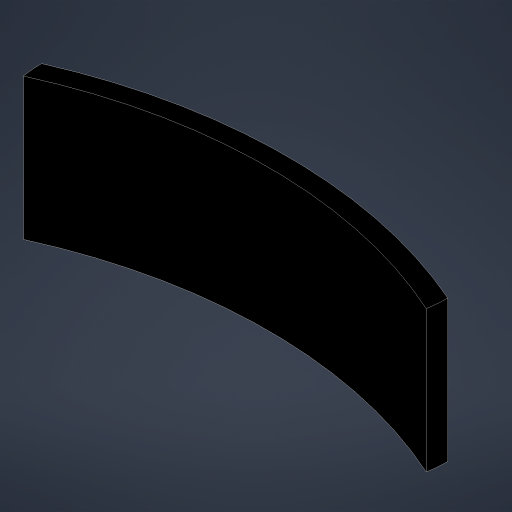
# Autodesk Inventor part: MettalringUnten_v3
Saved by Autodesk Inventor 2023.2 (Build 272271030, 271C)
## iProperties
Created: 2022-10-10
Part Number: MettalringUnten_v3
Material: Generic
Document SubType Name: Modeling
Designer: braun
Density: 1 g/cm^3
Appearance: Default
Author: braun
Autodesk Inventor part; units mm, degrees
ref_plane "YZ Plane" through (0, 0, 0) normal (1, 0, 0) x (0, 1, 0)
ref_plane "XZ Plane" through (0, 0, 0) normal (0, 1, 0) x (-1, 0, 0)
sketch "Sketch1" plane through (0, 0, 0) normal (0, 1, 0) x (-1, 0, 0)
  circle A0 centre (0, 0) radius 110 construction
  arc A1 (43.0581, -98.5) -> (-43.0581, -98.5) centre (0, 0) ccw
  line L0 (0, -107.5) -> (0, -98.5) construction
  line L1 (0, -98.5) -> (0, -73.5) construction
  line L2 (0, -98.5) -> (-43.0581, -98.5) construction
  line L3 (0, -98.5) -> (43.0581, -98.5) construction
  line L4 (43.0581, -98.5) -> (-43.0581, -98.5) construction
  line L5 (-18.0581, -73.5) -> (18.0581, -73.5)
  arc A2 (43.0581, -98.5) -> (18.0581, -73.5) centre (18.0581, -98.5) ccw
  arc A3 (-18.0581, -73.5) -> (-43.0581, -98.5) centre (-18.0581, -98.5) ccw
  line L6 (0, 107.5) -> (0, 97.5) construction
  line L7 (0, 97.5) -> (-22.5, 97.5) construction
  line L8 (-22.5, 97.5) -> (-22.5, 82.5) construction
  line L9 (22.5, 82.5) -> (22.5, 97.5) construction
  line L10 (22.5, 90) -> (-22.5, 90) construction
  line L11 (15, 97.5) -> (-15, 97.5)
  line L12 (-15, 82.5) -> (15, 82.5)
  arc A4 (15, 82.5) -> (15, 97.5) centre (15, 90) ccw
  arc A5 (-15, 97.5) -> (-15, 82.5) centre (-15, 90) ccw
  line L13 (22.5, 82.5) -> (17.5, 82.5) construction
  line L14 (17.5, 82.5) -> (17.5, 77.5) construction
  circle A6 centre (17.5, 77.5) radius 1.6
  circle A7 centre (-17.5, 77.5) radius 1.6
  line L15 (-58.336309, 79.549513) -> (-79.549513, 58.336309)
  arc A8 (-47.729708, 68.942911) -> (-58.336309, 79.549513) centre (-53.033009, 74.246212) ccw
  arc A9 (-79.549513, 58.336309) -> (-68.942911, 47.729708) centre (-74.246212, 53.033009) ccw
  line L16 (-68.942911, 47.729708) -> (-47.729708, 68.942911)
  circle A10 centre (-67.175144, 42.426407) radius 1.6
  circle A11 centre (-42.426407, 67.175144) radius 1.6
  line L17 (-97.5, 15) -> (-97.5, -15)
  arc A12 (-82.5, 15) -> (-97.5, 15) centre (-90, 15) ccw
  arc A13 (-97.5, -15) -> (-82.5, -15) centre (-90, -15) ccw
  line L18 (-82.5, -15) -> (-82.5, 15)
  circle A14 centre (-77.5, -17.5) radius 1.6
  circle A15 centre (-77.5, 17.5) radius 1.6
  line L19 (-79.549513, -58.336309) -> (-58.336309, -79.549513)
  arc A16 (-68.942911, -47.729708) -> (-79.549513, -58.336309) centre (-74.246212, -53.033009) ccw
  arc A17 (-58.336309, -79.549513) -> (-47.729708, -68.942911) centre (-53.033009, -74.246212) ccw
  line L20 (-47.729708, -68.942911) -> (-68.942911, -47.729708)
  circle A18 centre (-42.426407, -67.175144) radius 1.6
  circle A19 centre (-67.175144, -42.426407) radius 1.6
  line L21 (-15, -97.5) -> (15, -97.5)
  arc A20 (-15, -82.5) -> (-15, -97.5) centre (-15, -90) ccw
  arc A21 (15, -97.5) -> (15, -82.5) centre (15, -90) ccw
  line L22 (15, -82.5) -> (-15, -82.5)
  circle A22 centre (17.5, -77.5) radius 1.6
  circle A23 centre (-17.5, -77.5) radius 1.6
  line L23 (58.336309, -79.549513) -> (79.549513, -58.336309)
  arc A24 (47.729708, -68.942911) -> (58.336309, -79.549513) centre (53.033009, -74.246212) ccw
  arc A25 (79.549513, -58.336309) -> (68.942911, -47.729708) centre (74.246212, -53.033009) ccw
  line L24 (68.942911, -47.729708) -> (47.729708, -68.942911)
  circle A26 centre (67.175144, -42.426407) radius 1.6
  circle A27 centre (42.426407, -67.175144) radius 1.6
  line L25 (97.5, -15) -> (97.5, 15)
  arc A28 (82.5, -15) -> (97.5, -15) centre (90, -15) ccw
  arc A29 (97.5, 15) -> (82.5, 15) centre (90, 15) ccw
  line L26 (82.5, 15) -> (82.5, -15)
  circle A30 centre (77.5, 17.5) radius 1.6
  circle A31 centre (77.5, -17.5) radius 1.6
  line L27 (79.549513, 58.336309) -> (58.336309, 79.549513)
  arc A32 (68.942911, 47.729708) -> (79.549513, 58.336309) centre (74.246212, 53.033009) ccw
  arc A33 (58.336309, 79.549513) -> (47.729708, 68.942911) centre (53.033009, 74.246212) ccw
  line L28 (47.729708, 68.942911) -> (68.942911, 47.729708)
  circle A34 centre (42.426407, 67.175144) radius 1.6
  circle A35 centre (67.175144, 42.426407) radius 1.6
  line L29 (58.336309, -58.336309) -> (51.265242, -51.265242) construction
  line L30 (40.65864, -61.871843) -> (61.871843, -40.65864)
  arc A36 (40.65864, -61.871843) -> (44.52672, -89.539774) centre (53.033009, -74.246212) ccw
  arc A37 (89.539774, -44.52672) -> (61.871843, -40.65864) centre (74.246212, -53.033009) ccw
  line L31 (0, -73.5) -> (0, -66.5) construction
  arc A38 (44.52672, 89.539774) -> (40.65864, 61.871843) centre (53.033009, 74.246212) ccw
  line L32 (61.871843, 40.65864) -> (40.65864, 61.871843)
  arc A39 (61.871843, 40.65864) -> (89.539774, 44.52672) centre (74.246212, 53.033009) ccw
  arc A40 (-89.539774, 44.52672) -> (-61.871843, 40.65864) centre (-74.246212, 53.033009) ccw
  line L33 (-40.65864, 61.871843) -> (-61.871843, 40.65864)
  arc A41 (-40.65864, 61.871843) -> (-44.52672, 89.539774) centre (-53.033009, 74.246212) ccw
  arc A42 (-44.52672, -89.539774) -> (-40.65864, -61.871843) centre (-53.033009, -74.246212) ccw
  line L34 (-61.871843, -40.65864) -> (-40.65864, -61.871843)
  arc A43 (-61.871843, -40.65864) -> (-89.539774, -44.52672) centre (-74.246212, -53.033009) ccw
  arc A44 (89.539774, -44.52672) -> (89.539774, 44.52672) centre (0, 0) ccw
  arc A45 (44.52672, 89.539774) -> (-44.52672, 89.539774) centre (0, 0) ccw
  arc A46 (-89.539774, 44.52672) -> (-89.539774, -44.52672) centre (0, 0) ccw
  line L35 (43.0581, -98.5) -> (48.0581, -98.5) construction
  line L36 (48.0581, -98.5) -> (48.0581, -88.5) construction
  circle A47 centre (48.0581, -88.5) radius 1.6
  circle A48 centre (-48.0581, -88.5) radius 1.6
  line L37 (18.0581, -66.5) -> (-18.0581, -66.5)
  arc A49 (17.5, -66.5) -> (43.0581, -59.472383) centre (19.514525, -23.837671) ccw
  arc A50 (-44.52672, -58.003763) -> (-18.0581, -66.5) centre (-19.508856, -25.542168) ccw
  arc A51 (-48.0581, -88.5) -> (-42.426407, -67.175144) centre (-60.43967, -73.824078) ccw construction
  arc A52 (-48.0581, -88.5) -> (-42.426407, -67.175144) centre (-60.43967, -73.824078) ccw construction
  arc A53 (-44.936716, -92.199789) -> (-37.885276, -65.498953) centre (-60.43967, -73.824078) ccw
  arc A54 (-51.179485, -84.800211) -> (-46.967537, -68.851335) centre (-60.43967, -73.824078) ccw
  arc A55 (-51.179485, -84.800211) -> (-44.936716, -92.199789) centre (-48.0581, -88.5) ccw
  arc A56 (-37.885276, -65.498953) -> (-46.967537, -68.851335) centre (-42.426407, -67.175144) ccw
  line L38 (42.426407, 67.175144) -> (67.175144, 42.426407) construction
  line L39 (45.961941, 70.710678) -> (70.710678, 45.961941)
  line L40 (63.63961, 38.890873) -> (38.890873, 63.63961)
  arc A57 (45.961941, 70.710678) -> (38.890873, 63.63961) centre (42.426407, 67.175144) ccw
  arc A58 (63.63961, 38.890873) -> (70.710678, 45.961941) centre (67.175144, 42.426407) ccw
  line L41 (-42.426407, 67.175144) -> (-67.175144, 42.426407) construction
  line L42 (-45.961941, 70.710678) -> (-70.710678, 45.961941)
  line L43 (-63.63961, 38.890873) -> (-38.890873, 63.63961)
  arc A59 (-38.890873, 63.63961) -> (-45.961941, 70.710678) centre (-42.426407, 67.175144) ccw
  arc A60 (-70.710678, 45.961941) -> (-63.63961, 38.890873) centre (-67.175144, 42.426407) ccw
  line L44 (-42.426407, 67.175144) -> (42.426407, 67.175144) construction
  line L45 (-42.426407, 62.175144) -> (42.426407, 62.175144)
  line L46 (42.426407, 72.175144) -> (-42.426407, 72.175144)
  arc A61 (-42.426407, 72.175144) -> (-42.426407, 62.175144) centre (-42.426407, 67.175144) ccw
  arc A62 (42.426407, 62.175144) -> (42.426407, 72.175144) centre (42.426407, 67.175144) ccw
  line L47 (37.025198, 67.175144) -> (33.025198, 67.175144) construction
  line L48 (33.025198, 67.175144) -> (32.025198, 67.175144) construction
  line L49 (31.025198, 70.425144) -> (31.025198, 63.925144)
  line L50 (31.025198, 63.925144) -> (33.025198, 63.925144)
  line L51 (33.025198, 63.925144) -> (33.025198, 70.425144)
  line L52 (33.025198, 70.425144) -> (31.025198, 70.425144)
  line L53 (31.025198, 70.425144) -> (33.025198, 63.925144) construction
  line L54 (31.025198, 63.925144) -> (33.025198, 70.425144) construction
  line L55 (0, 67.175144) -> (0, 56.50884) construction
  line L56 (-31.025198, 70.425144) -> (-31.025198, 63.925144)
  line L57 (-31.025198, 63.925144) -> (-33.025198, 63.925144)
  line L58 (-33.025198, 63.925144) -> (-33.025198, 70.425144)
  line L59 (-33.025198, 70.425144) -> (-31.025198, 70.425144)
  arc A63 (-43.0581, -98.5) -> (43.0581, -98.5) centre (0, 0) ccw
  line L60 (0, -107.5) -> (0, -103.5)
  arc A64 (-41.455938, -94.834884) -> (41.455938, -94.834884) centre (0, 0) ccw
  arc A65 (41.455938, -94.834884) -> (42.699608, -94.281459) centre (0, 0) ccw
  arc A66 (-42.699608, -94.281459) -> (-41.455938, -94.834884) centre (0.000004, 0.000008) ccw
  point P0 (0, 90)
  point P1 (-45.961941, 70.710678)
  point P2 (-82.5, 17.5)
  point P3 (-70.710678, -45.961941)
  point P4 (-17.5, -82.5)
  point P5 (45.961941, -70.710678)
  point P6 (82.5, -17.5)
  point P7 (70.710678, 45.961941)
  point P8 (35.715922, -76.769806)
  point P9 (-37.90233, -65.453455)
  point P10 (-39.097126, -63.661261)
  point P11 (-46.422064, -70.704261)
  point P12 (-46.867306, -78.516354)
  point P13 (0, -44.52672)
  point P14 (0, 35.701561)
  point P15 (54.800776, 54.800776)
  point P16 (-54.800776, 54.800776)
  point P17 (40.355339, 62.175144)
  point P18 (40.65864, 61.871843)
  point P19 (-47.729708, 68.942911)
  point P20 (-68.942911, 47.729708)
  point P21 (-61.871843, 40.65864)
  point P22 (-40.355339, 62.175144)
  dimension "d0" = 220
  dimension "d1" = 215
  dimension "d2" = 9
  dimension "d3" = 25
  dimension "d4" = 10
  dimension "d5" = 22.5
  dimension "d6" = 15
  dimension "d7" = 45
  dimension "d8" = 5
  dimension "d9" = 5
  dimension "d10" = 3.2
  dimension "d15" = 86.1162
  dimension "d16" = 45
  dimension "d19" = 360
  dimension "d22" = 10
  dimension "d23" = 7
  dimension "d26" = 360
  dimension "d33" = 5
  dimension "d34" = 10
  dimension "d35" = 3.2
  dimension "d68" = 4
  dimension "d69" = 1
  dimension "d70" = 6.5
  dimension "d71" = 2
  dimension "d123" = 4
  constraints: 132 end point, 107 point on circle, 67 centre point, 24 tangent, 23 point on line, 10 midpoint, 6 parallel, 6 symmetric about line, 5 coincident, 5 vertical, 4 perpendicular, 3 horizontal, 2 concentric, 1 collinear, 160 other
  measures "d0" diameter of A0
  measures "d1" diameter of A1
  measures "d2" distance of L0.start L0.end
  measures "d3" distance of L0.end L1.end
  measures "d4" distance of L6.start L6.end
  measures "d5" distance of L6.end L7.end
  measures "d6" distance of L7.end L8.end
  measures "d7" distance of L8.end L9.start
  measures "d8" distance of L9.start L13.end
  measures "d9" distance of L13.end L14.end
  measures "d10" diameter of A6
  measures "d15" distance of L3.end L2.end
  measures "d16" distance of L10.start L10.end
  measures "d22" distance of L29.start L29.end
  measures "d23" distance of L1.end L31.end
  measures "d33" distance of L3.end L35.end
  measures "d34" distance of L35.end L36.end
  measures "d35" diameter of A47
  measures "d68" distance of L47.start L47.end
  measures "d69" distance of L47.end L48.end
  measures "d70" distance of L49.start L49.end
  measures "d71" distance of L50.end L49.end
  measures "d123" distance of L0.start L60.end
ref_plane "Work Plane4" through (0, 0, -44.52672) normal (1, 0, 0) x (0, 0.9903099, -0.1388753)
extrude "Extrusion13" add sketch "Sketch1" against normal blind 30 contours A63 L60 A64 A65 A2 | A3 A66 A64 L60 A63
body "Solid4"
